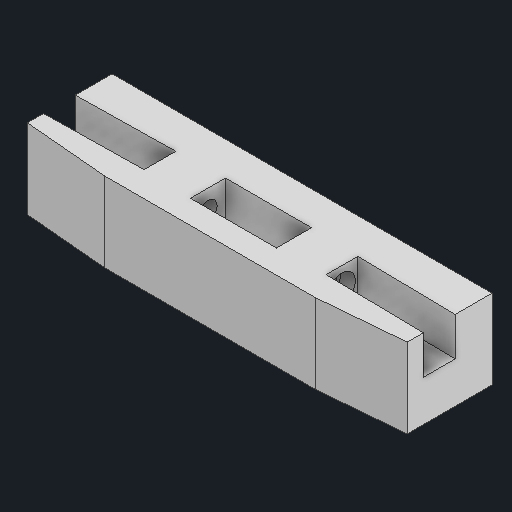
# Autodesk Inventor part: Camera_Clip
Saved by Autodesk Inventor 2024 (Build 280153000, 153)
## iProperties
Created: 2025-09-25
Part Number: Camera_Clip
Material: Generic
Document SubType Name: Modeling
Designer: kevin
Density: 1 g/cm^3
Appearance: Default
Author: kevin
Autodesk Inventor part; units mm, degrees
ref_plane "YZ Plane" through (0, 0, 0) normal (1, 0, 0) x (0, 1, 0)
ref_plane "XZ Plane" through (0, 0, 0) normal (0, 1, 0) x (-1, 0, 0)
ref_plane "XY Plane" through (0, 0, 0) normal (0, 0, 1) x (1, 0, 0)
sketch "Sketch1" plane through (0, 0, 0) normal (0, 1, 0) x (-1, 0, 0)
  line L0 (-10.4458, -2.7323) -> (-10.4458, 5.0177)
  line L1 (-10.4458, 5.0177) -> (9.7542, 5.0177)
  line L2 (9.7542, 5.0177) -> (9.7542, -2.7323)
  line L3 (9.7542, -2.7323) -> (-10.4458, -2.7323)
  line L4 (46.0042, -11.3323) -> (-46.6958, -11.3323)
  line L5 (46.0042, 9.3619) -> (46.0042, -11.3323)
  line L6 (25.3638, 11.1677) -> (46.0042, 9.3619)
  line L7 (-26.0554, 11.1677) -> (25.3638, 11.1677)
  line L8 (-46.6958, 9.3619) -> (-26.0554, 11.1677)
  line L9 (-46.6958, 9.3619) -> (-46.6958, -11.3323)
  line L10 (10.1542, 5.4177) -> (-10.8458, 5.4177)
  line L11 (-10.8458, 5.4177) -> (-10.8458, -3.1323)
  line L12 (-10.8458, -3.1323) -> (10.1542, -3.1323)
  line L13 (10.1542, -3.1323) -> (10.1542, 5.4177)
  line L14 (-10.8458, 5.0177) -> (-22.5458, 5.0177)
  line L15 (-22.5458, 5.0177) -> (-22.5458, -2.7323)
  line L16 (-22.5458, -2.7323) -> (-10.8458, -2.7323)
  line L17 (-0.3458, 5.0177) -> (-0.3458, 1.5521) construction
  line L18 (-22.5458, 5.0177) -> (-46.6958, 5.4177)
  line L19 (-22.5458, -2.7323) -> (-46.6958, -2.3323)
  line L20 (21.8542, 5.0177) -> (46.0042, 5.4177)
  line L21 (21.8542, -2.7323) -> (46.0042, -2.3323)
  line L22 (21.8542, -2.7323) -> (10.1542, -2.7323)
  line L23 (21.8542, 5.0177) -> (21.8542, -2.7323)
  line L24 (10.1542, 5.0177) -> (21.8542, 5.0177)
  point P0 (0, 0)
  dimension "d0" = 0.4
  dimension "d1" = 11.7
  constraints: 50 end point, 6 symmetric about line, 4 point on line, 2 perpendicular, 1 horizontal, 1 midpoint, 1 parallel, 1 vertical, 3 other
  measures "d0" distance between parallel lines of L1 L10
  measures "d1" distance of L14.start L14.end
extrude "Extrusion1" add sketch "Sketch1" along normal blind 9.398 contours L4 L9 L19 L16 L11 L12 L13 L22 L21 L5 | L20 L24 L13 L10 L11 L14 L18 L9 L8 L7 L6 L5 | L22 L13 L24 L23 | L15 L14 L11 L16
sketch "Sketch2" plane through (0, 0, 0) normal (0, -1, 0) x (1, 0, 0)
  line L0 (-21.8542, 5.0177) -> (-46.0042, 5.4177) projected
  line L1 (-21.8542, -2.7323) -> (-21.8542, 5.0177) projected
  line L2 (-46.0042, -2.3323) -> (-21.8542, -2.7323) projected
  line L3 (-46.0042, -11.3323) -> (-46.0042, -2.3323) projected
  line L4 (46.6958, -11.3323) -> (-46.0042, -11.3323) projected
  line L5 (46.6958, -2.3323) -> (46.6958, -11.3323) projected
  line L6 (22.5458, -2.7323) -> (46.6958, -2.3323) projected
  line L7 (22.5458, 5.0177) -> (22.5458, -2.7323) projected
  line L8 (46.6958, 5.4177) -> (22.5458, 5.0177) projected
  line L9 (46.6958, 9.3619) -> (46.6958, 5.4177) projected
  line L10 (26.0554, 11.1677) -> (46.6958, 9.3619) projected
  line L11 (-25.3638, 11.1677) -> (26.0554, 11.1677) projected
  line L12 (-46.0042, 9.3619) -> (-25.3638, 11.1677) projected
  line L13 (-46.0042, 5.4177) -> (-46.0042, 9.3619) projected
  line L14 (-10.1542, 5.4177) -> (-10.1542, -3.1323) projected
  line L15 (10.8458, 5.4177) -> (-10.1542, 5.4177) projected
  line L16 (10.8458, -3.1323) -> (10.8458, 5.4177) projected
  line L17 (-10.1542, -3.1323) -> (10.8458, -3.1323) projected
  line L18 (46.6958, 5.4177) -> (46.6958, -2.3323)
  line L19 (-46.0042, 5.4177) -> (-46.0042, -2.3323)
  point P0 (0, 0)
  constraints: 4 end point, 1 parallel, 1 vertical
extrude "Extrusion2" add sketch "Sketch2" along normal blind 10 contours L1 L2 L19 L0 | L0 L13 L12 L11 L10 L9 L8 L7 L6 L5 L4 L3 L2 L1 | L6 L7 L8 L18 | L15 L16 L17 L14
sketch "Sketch3" plane through (0, -10, 0) normal (0, -1, 0) x (1, 0, 0)
  line L0 (46.6958, 9.3619) -> (26.0554, 11.1677) projected
  line L1 (26.0554, 11.1677) -> (-25.3638, 11.1677) projected
  line L2 (-25.3638, 11.1677) -> (-46.0042, 9.3619) projected
  line L3 (-46.0042, 9.3619) -> (-46.0042, -11.3323) projected
  line L4 (-46.0042, -11.3323) -> (46.6958, -11.3323) projected
  line L5 (46.6958, -11.3323) -> (46.6958, 9.3619) projected
  line L6 (46.6958, -0.9852) -> (-46.0042, -0.9852) construction
  circle A0 centre (34.6958, -0.9852) radius 2.1
  line L7 (0, 0) -> (0, -4.846) construction
  circle A1 centre (-34.6958, -0.9852) radius 2.1
  circle A2 centre (0, -0.9852) radius 2.1
  dimension "d6" = 4.2
  dimension "d7" = 12
  dimension "d10" = 4.2
  constraints: 4 end point, 3 centre point, 3 point on line, 2 midpoint, 1 symmetric about line, 1 other
  measures "d6" diameter of A0
  measures "d7" distance from line of L5 A0.centre
  measures "d10" diameter of A2
extrude "Extrusion3" cut sketch "Sketch3" against normal blind 8 contours A0 | A1 | A2
sketch "Sketch4" plane through (22.5458, 9.398, 5.0177) normal (1, 0, 0) x (0, 0, -1)
  circle A0 centre (3.875, -4.85) radius 2.25 projected
  point P0 (5.0177, -9.398)
extrude "Extrusion4" cut sketch "Sketch4" along normal blind 8 and the other way blind 50.0253
sketch "Sketch5" plane through (22.5458, 9.398, 5.0177) normal (1, 0, 0) x (0, 0, -1)
  circle A0 centre (3.875, -4.85) radius 2.25 projected
  line L0 (0, -9.398) -> (7.75, -9.398) projected
  line L1 (7.75, -9.398) -> (7.75, 0) projected
  line L2 (0, 0) -> (7.75, 0) projected
  line L3 (0, -9.398) -> (0, 0) projected
  circle A1 centre (3.875, -4.85) radius 3.3
  point P0 (5.0177, -9.398)
  dimension "d15" = 6.6
  constraints: 1 centre point, 1 coincident
  measures "d15" diameter of A1
extrude "Extrusion5" cut sketch "Sketch5" against normal blind 3.5 contours A0 | A1
mirror "Mirror1" about plane through (0, 0, 0) normal (1, 0, 0) of "Extrusion5"
body "Solid1"
